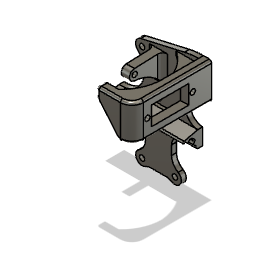
Camera_Pivot v57 (Autodesk Fusion 360 design; units mm, degrees)
Autodesk Fusion 360 part; units mm, degrees
note: some values were not read from the file. Set by a fixed rule: which sketch regions a step uses.
sketch "Skizze1" plane through (0, 0, 0) normal (0, 0, 1) x (1, 0, 0)
  circle A0 centre (-10, 0) radius 1.6
  circle A1 centre (16, 0) radius 1.6
  line L0 (0, 0) -> (0, 50.3542) construction
  arc A2 (-10.8907, 3.8996) -> (-12.8166, -2.8402) centre (-10, 0) ccw
  circle A3 centre (0, -22) radius 1.6
  arc A4 (-24, -27) -> (-12.8166, -2.8402) centre (-22.7861, -12.8936) ccw
  line L1 (24.5, -11) -> (24.5, 11)
  arc A5 (24.5, 11) -> (16, 10.0416) centre (24.5, -27.1726) ccw
  line L2 (-10, 0) -> (16, 0) construction
  line L3 (-10.8907, 3.8996) -> (16, 10.0416)
  arc A6 (24.5, -11) -> (24, -27) centre (24.5, -19.0078) ccw
  line L4 (24.5, 11) -> (33, 11) construction
  line L5 (24.5, -11) -> (33, -11) construction
  line L6 (-24, -27) -> (24, -27) construction
  line L7 (24, -27) -> (24, -37)
  line L8 (-24, -37) -> (-24, -27)
  line L9 (0, 0) -> (0, -27) construction
  circle A7 centre (-10, -59) radius 1.6
  circle A8 centre (10, -59) radius 1.6
  arc A9 (-12, -55.5359) -> (-6.8775, -61.5) centre (-10, -59) ccw
  arc A10 (6.8775, -61.5) -> (12, -55.5359) centre (10, -59) ccw
  line L10 (24, -37) -> (8, -37)
  line L11 (-8, -37) -> (-24, -37)
  line L12 (8, -37) -> (-8, -37) construction
  line L13 (-8, -37) -> (-8, -48.6077)
  arc A11 (-12, -55.5359) -> (-8, -48.6077) centre (-16, -48.6077) ccw
  arc A12 (8, -48.6077) -> (12, -55.5359) centre (16, -48.6077) ccw
  line L14 (8, -48.6077) -> (8, -37)
  line L15 (-6.8775, -61.5) -> (6.8775, -61.5)
  dimension "d1" = 3.2
  dimension "d3" = 4
  dimension "d22" = 22
  dimension "d23" = 11
  dimension "d57" = 10
  dimension "d58" = 22
  dimension "d59" = 24.5
  dimension "d60" = 16
  dimension "d62" = 48
  dimension "d63" = 10
  dimension "d81" = 5
  dimension "d83" = 20
  dimension "d84" = 22
  dimension "d85" = 4
  dimension "d86" = 16
  dimension "d87" = 8
  dimension "d90" = 2.5
  constraint coincident L0.start L9.start
  constraint vertical L0
  constraint concentric A0 A2
  constraint equal A1 A3
  constraint tangent A2 A4
  constraint vertical L1
  constraint coincident L1.end A5.start
  constraint coincident A0.centre A2.centre
  constraint coincident A1.centre L2.end
  constraint coincident L0.start L2
  constraint tangent A5 L3
  constraint tangent A2 L3
  constraint tangent A5 L4
  constraint perpendicular L1 L4
  constraint vertical A1.centre A5.end
  constraint perpendicular L1 L5
  constraint tangent A6 L5
  constraint equal A0 A1
  constraint horizontal L2
  constraint horizontal L6
  constraint vertical L7
  constraint horizontal L10
  constraint vertical L8
  constraint midpoint L6 L9.end
  constraint coincident A3.centre L9
  constraint vertical L9
  constraint symmetric L9 A7 A8
  constraint equal A3 A8
  constraint coincident L11.start L10
  constraint concentric A8 A10
  constraint concentric A7 A9
  constraint horizontal L11
  constraint perpendicular L12 L13
  constraint tangent L13 A11
  constraint tangent A10 A12
  constraint symmetric L9 L13 L14
  constraint equal L13 L14
  constraint symmetric L9 A11 A12
  constraint tangent A9 A11
  constraint horizontal L15
  constraint coincident A10.start L15.end
  measures "d1" diameter of A1
  measures "d3" radius of A2
  measures "d22" distance of L1.end L1.start
  measures "d23" vertical distance of A1.centre L1.end
  measures "d57" distance of L0.start A0.centre
  measures "d58" distance of A3.centre L2
  measures "d59" distance of L0 L1
  measures "d60" distance of L0.start A1.centre
  measures "d62" distance of A4.start A6.end
  measures "d63" distance of A6.end L7.end
  measures "d81" distance of A3.centre L6
  measures "d83" distance of A7.centre A8.centre
  measures "d84" distance of A8.centre L10
  measures "d85" radius of A10
  measures "d86" distance of L11.start L10.end
  measures "d87" radius of A12
  measures "d90" distance of A8.centre L15
extrude "Extrusion1" add sketch "Skizze1" along normal blind 3
sketch "Skizze2" plane through (0, 0, 0) normal (1, 0, 0) x (0, 0, -1)
  circle A0 centre (-20, 0) radius 1.575
  line L0 (-3, 3.8996) -> (-20.1236, 3.2476)
  line L1 (0, 0) -> (-20, 0) construction
  arc A1 (-20.1236, 3.2476) -> (-20.2376, -3.2413) centre (-20, 0) ccw
  line L2 (-3, -27.0521) -> (-3, -2.8402)
  line L3 (-3, 3.8996) -> (-3, -2.8402)
  arc A2 (-3, -13.1004) -> (-20.2376, -3.2413) centre (-21.9191, -26.1798) ccw
  dimension "d6" = 3.15
  dimension "d7" = 6.5
  dimension "d8" = 20
  dimension "d14" = 23
  dimension "d15" = 17
  constraint concentric A0 A1
  constraint tangent L0 A1
  constraint coincident L1.start origin
  constraint coincident A0.centre L1.end
  constraint horizontal L1
  constraint coincident L2 A2.start
  constraint tangent A1 A2
  constraint coincident L0.start L3.start
  measures "d6" diameter of A0
  measures "d7" diameter of A1
  measures "d8" distance of L1.start A0.centre
  measures "d14" radius of A2
  measures "d15" distance of L0.start A2.start
extrude "Extrusion2" add sketch "Skizze2" along normal mid plane 5
fillet "Abrundung1" radius 3 2 edges at (2.5, -4.6004, 3) (-2.5, -4.6004, 3)
sketch "Skizze3" plane through (24.5, 0, 0) normal (1, 0, 0) x (0, 0, -1)
  line L0 (0, -11) -> (0, 11)
  line L1 (0, 11) -> (-3, 11)
  line L2 (-3, 11) -> (-3, -11)
  line L3 (-3, -11) -> (0, -11)
  line L4 (-3, 11) -> (-41.75, 11)
  line L5 (-41.75, -11) -> (-3, -11)
  line L6 (-3, 0) -> (-64.357, 0) construction
  line L7 (-36.75, 5.75) -> (-14, 5.75)
  line L8 (-14, 5.75) -> (-14, -5.75)
  line L9 (-14, -5.75) -> (-36.75, -5.75)
  line L10 (-36.75, -5.75) -> (-36.75, 5.75)
  circle A0 centre (-39.25, 0) radius 1.6
  circle A1 centre (-11.5, 0) radius 1.6
  line L11 (-39.25, 4.0803) -> (-39.25, -4.0803) construction
  line L12 (-41.75, 11) -> (-41.75, -11)
  dimension "d25" = 11.5
  dimension "d26" = 27.75
  dimension "d27" = 3.2
  dimension "d28" = 3.2
  dimension "d29" = 2.5
  dimension "d30" = 2.5
  dimension "d33" = 11.5
  dimension "d39" = 2.5
  constraint coincident L1.end L2.start
  constraint coincident L2.end L3.start
  constraint midpoint L2 L6.start
  constraint perpendicular L2 L6
  constraint horizontal L7
  constraint vertical L8
  constraint horizontal L9
  constraint vertical L10
  constraint symmetric L6 L7 L9
  constraint coincident L6 A0.centre
  constraint coincident L6 A1.centre
  constraint symmetric L4 L5 L6
  constraint coincident A0.centre L11
  constraint vertical L11
  constraint horizontal L5
  constraint perpendicular L5 L12
  measures "d25" distance of L7.end L8.end
  measures "d26" distance of A0.centre A1.centre
  measures "d27" diameter of A0
  measures "d28" diameter of A1
  measures "d29" distance of L10 A0.centre
  measures "d30" distance of L8 A1.centre
  measures "d33" distance of origin A1.centre
  measures "d39" distance of A0.centre L12
extrude "Extrusion3" add sketch "Skizze3" along normal blind 5
sketch "Skizze4" plane through (0, 5.75, 0) normal (0, -1, 0) x (1, 0, 0)
  line L0 (24.5, 36.75) -> (24.5, 14)
  line L1 (24.5, 14) -> (29.5, 14)
  line L2 (29.5, 14) -> (29.5, 36.75)
  line L3 (29.5, 36.75) -> (24.5, 36.75)
  line L4 (-5.5, 3) -> (5.5, 3)
  line L5 (16.4922, 3) -> (24.5, 3)
  line L6 (24.5, 3) -> (16, 3)
  line L7 (16, 3) -> (-10.8907, 3)
  line L8 (-10.8907, 3) -> (-14, 3)
  line L9 (-24, 3) -> (-8.6276, 3)
  line L10 (-11.6, 3) -> (-8.4, 3)
  line L11 (14.4, 3) -> (17.6, 3)
  line L12 (-1.6, 3) -> (1.6, 3)
  line L13 (24.5, 40.85) -> (24.5, 37.65)
  line L14 (24.5, 36.75) -> (24.5, 14)
  line L15 (24.5, 14) -> (24.5, 36.75)
  line L16 (24.5, 13.1) -> (24.5, 9.9)
  arc A0 (10.7456, 3) -> (24.5, 25.375) centre (-5.3558, 28.313) ccw
  line L17 (24.5, 3) -> (24.5, 41.75)
  line L18 (24.5, 41.75) -> (24.5, 3)
  line L19 (5.5, 3) -> (-5.5, 3)
  line L20 (-6.8775, 3) -> (-14, 3)
  line L21 (14, 3) -> (6.8775, 3)
  line L22 (8, 3) -> (24, 3)
  line L23 (-24, 3) -> (-8, 3)
  line L24 (8.4, 3) -> (11.6, 3)
  line L25 (-11.6, 3) -> (-8.4, 3)
  line L26 (8, 3) -> (12, 3)
  line L27 (-12, 3) -> (-8, 3)
  line L28 (-6.8775, 3) -> (6.8775, 3)
  dimension "d38" = 30
  constraint coincident L5 A0.start
  constraint midpoint L14 A0.end
  measures "d38" radius of A0
extrude "Extrusion8" add sketch "Skizze4" against normal blind 2.5 contours L0 L5 L6 L7 L11 L14 L15 L16 A0 L17 L18 L21 L22 L24 L26
extrude "Extrusion4" add sketch "Skizze4" against normal blind 2.5 contours L0 L5 L6 L7 L11 L14 L15 L16 A0 L17 L18 L21 L22 L24 L26
sketch "Skizze5" plane through (0, 11, 0) normal (0, 1, 0) x (-1, 0, 0)
  line L0 (-24.5, 0) -> (-24.5, 3)
  line L1 (-24.5, 3) -> (-24.5, 41.75)
  line L2 (-24.5, 41.75) -> (-29.5, 41.75)
  line L3 (-29.5, 41.75) -> (-29.5, 0)
  line L4 (-29.5, 0) -> (-24.5, 0)
  arc A0 (-22.5, 43.75) -> (-24.5, 41.75) centre (-22.5, 41.75) ccw
  line L5 (-22.5, 43.75) -> (-8, 43.75)
  line L6 (-8, 43.75) -> (-8, 48.75)
  line L7 (-8, 48.75) -> (-22.5, 48.75)
  arc A1 (-22.5, 48.75) -> (-29.5, 41.75) centre (-22.5, 41.75) ccw
  arc A2 (-16.5, 43.75) -> (-24.5, 25.375) centre (0.6025, 25.375) ccw
  line L8 (-24.5, 25.375) -> (-24.5, 19) construction
  point P0 (-24.5, 25.375)
  dimension "d41" = 8
  dimension "d42" = 2
  dimension "d55" = 8
  constraint coincident L1.end L2.start
  constraint tangent L1 A0
  constraint tangent A0 L5
  constraint perpendicular L5 L6
  constraint perpendicular L6 L7
  constraint coincident L2.end L3.start
  constraint tangent L7 A1
  constraint concentric A0 A1
  constraint horizontal L5
  constraint coincident L5 A2.start
  constraint coincident L1 L8.end
  constraint parallel L1 L8
  constraint tangent A2 L8
  measures "d41" distance of origin L6
  measures "d42" radius of A0
  measures "d55" horizontal distance of L1.end A2.start
extrude "Extrusion5" add sketch "Skizze5" against normal blind 22 contours L2 A0 L5 L6 L7 A1
extrude "Extrusion6" add sketch "Skizze5" against normal blind 3 contours L1 A0 L5 A2
sketch "Skizze6" plane through (0, 11, 0) normal (0, 1, 0) x (-1, 0, 0)
sketch "Skizze7" plane through (0, 0, 48.75) normal (0, 0, 1) x (1, 0, 0)
  line L0 (22.5, 11) -> (8, 11)
  line L1 (8, 11) -> (8, -11)
  line L2 (8, -11) -> (22.5, -11)
  line L3 (22.5, -11) -> (22.5, 11)
  line L4 (8, 9.5) -> (8, 5.5649)
  arc A0 (8, 5.5649) -> (8.9306, 3) centre (12, 5.5649) ccw
  line L5 (8.9306, 3) -> (19.4306, -9.5649)
  arc A1 (19.4306, -9.5649) -> (22.5, -11) centre (22.5, -7) ccw
  line L6 (22.5, -11) -> (29.5, -11)
  arc A2 (9.5, 11) -> (8, 9.5) centre (9.5, 9.5) ccw
  line L7 (9.5, 11) -> (22.5, 11)
  dimension "d47" = 1.5
  dimension "d48" = 4
  dimension "d49" = 4
  dimension "d50" = 8
  constraint coincident L1 L4.end
  constraint tangent L4 A0
  constraint coincident L2.end L3.start
  constraint tangent L5 A1
  constraint tangent A1 L6
  constraint tangent A0 L5
  constraint coincident L1 L4.start
  constraint coincident L0 A2.start
  constraint tangent L4 A2
  constraint coincident L0.start L3.end
  constraint tangent A2 L7
  measures "d47" radius of A2
  measures "d48" radius of A0
  measures "d49" radius of A1
  measures "d50" distance of A0.end L7
extrude "Extrusion7" cut sketch "Skizze7" against normal blind 7 contours L0 L1 A2 | L1 L2 A0 L5 A1
sketch "Skizze8" plane through (-24, 0, 0) normal (-1, 0, 0) x (0, 0, 1)
  line L0 (0, -27) -> (0, -37)
  line L1 (3, -37) -> (3, -27)
  line L2 (3, -27) -> (0, -27)
  line L3 (12.8501, -29.3042) -> (3, -27)
  line L4 (3, -37) -> (4.576, -35.7687)
  line L5 (4.576, -35.7687) -> (3.9604, -34.9807)
  line L6 (3.9604, -34.9807) -> (5.7334, -33.5954)
  line L7 (5.7334, -33.5954) -> (4.1942, -31.6254)
  line L8 (4.1942, -31.6254) -> (7.3463, -29.1628)
  line L9 (7.3463, -29.1628) -> (8.8854, -31.1328)
  line L10 (8.8854, -31.1328) -> (10.6585, -29.7475)
  line L11 (10.6585, -29.7475) -> (11.2741, -30.5356)
  line L12 (11.2741, -30.5356) -> (12.8501, -29.3042)
  line L13 (0, -37) -> (3, -37)
  dimension "d69" = 4
  dimension "d70" = 8.5
  dimension "d71" = 1
  dimension "d73" = 2.5
  dimension "d74" = 52
  dimension "d82" = 2
  constraint coincident L1.end L2.start
  constraint coincident L1.start L4.start
  constraint perpendicular L4 L5
  constraint perpendicular L5 L6
  constraint perpendicular L6 L7
  constraint perpendicular L7 L8
  constraint perpendicular L8 L9
  constraint perpendicular L9 L10
  constraint perpendicular L10 L11
  constraint parallel L10 L12
  constraint equal L6 L10
  constraint equal L4 L12
  constraint collinear L4 L12
  constraint collinear L6 L10
  measures "d69" distance of L7.end L8.end
  measures "d70" distance of L5 L11
  measures "d71" distance of L10.end L11.end
  measures "d73" distance of L8.end L9.end
  measures "d74" angle of L1 L4
  measures "d82" distance of L1.start L4.end
extrude "Extrusion9" add sketch "Skizze8" against normal blind 48 contours L1 L3 L4 L5 L6 L7 L8 L9 L10 L11 L12
sketch "Skizze9" plane through (0, 0, 3) normal (0, 0, 1) x (1, 0, 0)
  line L0 (-21.5723, -27) -> (24, -27)
  arc A0 (24.5, -11) -> (24, -27) centre (24.5, -19.0078) ccw
  line L1 (24.5, -11) -> (24.5, 5.75)
  line L2 (24.5, 5.75) -> (10.7456, 5.75)
  line L3 (10.7456, 5.75) -> (10.7456, 8.25)
  line L4 (16, 10.0416) -> (-10.8907, 3.8996)
  arc A1 (-10.8907, 3.8996) -> (-12.8166, -2.8402) centre (-10, 0) ccw
  arc A2 (-21.5723, -27) -> (-12.8166, -2.8402) centre (-22.7861, -12.8936) ccw
  line L5 (-5.5, 3.8996) -> (5.5, 3.8996)
  line L6 (5.5, 3.8996) -> (5.5, -13.1004)
  line L7 (5.5, -13.1004) -> (-5.5, -13.1004)
  line L8 (-5.5, -13.1004) -> (-5.5, 3.8996)
  circle A3 centre (-10, 0) radius 1.6
  circle A4 centre (16, 0) radius 1.6
  circle A5 centre (0, -22) radius 1.6
  line L9 (-6, -27) -> (6, -27)
  line L10 (6, -27) -> (6, -25)
  line L11 (6, -25) -> (-6, -25)
  line L12 (-6, -25) -> (-6, -27)
  line L13 (0, 0) -> (0, -25) construction
  line L14 (6, -37) -> (-6, -37)
  line L15 (-6, -37) -> (-6, -39)
  line L16 (-6, -39) -> (6, -39)
  line L17 (6, -39) -> (6, -37)
  line L18 (8, -37) -> (24, -37)
  line L19 (10.7456, 8.25) -> (24.5, 8.25)
  line L20 (24.5, 8.25) -> (24.5, 11)
  arc A6 (24.5, 11) -> (16, 10.0416) centre (24.5, -27.1726) ccw
  dimension "d75" = 2
  dimension "d76" = 12
  dimension "d91" = 2
  dimension "d92" = 12
  constraint horizontal L9
  constraint vertical L10
  constraint horizontal L11
  constraint vertical L12
  constraint coincident L0 L9.start
  constraint coincident L13.start origin
  constraint midpoint L11 L13.end
  constraint vertical L13
  constraint horizontal L16
  constraint vertical L17
  constraint horizontal L14
  constraint vertical L15
  constraint coincident L14.start L18
  constraint collinear L10 L17
  measures "d75" distance of L9.end L10.end
  measures "d76" distance of L10.end L11.end
  measures "d91" distance of L16.end L14.start
  measures "d92" distance of L14.end L14.start
extrude "Extrusion10" cut sketch "Skizze9" against normal blind 8 contours L0 L9 L10 L11 L12 | L14 L15 L16 L17
fillet "Abrundung2" radius 0.75 3 edges at (0, -29.3042, 12.8501) (0, -35.7687, 4.576) (0, -30.5356, 11.2741)
fillet "Abrundung3" radius 6 4 edges at (-8, -37, 1.5) (8, -37, 1.5) (-6.8775, -61.5, 1.5) (6.8775, -61.5, 1.5)
fillet "Abrundung4" radius 1.5 10 edges at (29.5, 11, 20.875) (27.4497, 11, 46.6997) (16, 11, 48.75) (8.4393, 10.5607, 48.75) (8, 7.5325, 48.75) (8.2398, 4.2007, 48.75) (14.1806, -3.2825, 48.75) (20.8059, -10.6235, 48.75) (27.4497, -11, 46.6997) (29.5, -11, 20.875)
fillet "Abrundung5" radius 1 2 edges at (0, -29.1628, 7.3463) (0, -31.6254, 4.1942)
